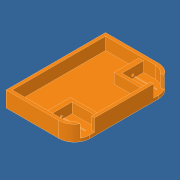
# Autodesk Inventor part: P1794_001
Saved by Autodesk Inventor 2019 (Build 230136000, 136)
## iProperties
Created: 2019-04-29
Part Number: P1794_001
Material: PLA
Document SubType Name: Modeling
Designer: Joan.MAILLARD
Density: 1.25 g/cm^3
Appearance: Orange
Project: P1704 Manette
Description: Bas manette
Author: Joan.MAILLARD
Title: P1704_001_basManette
Autodesk Inventor part; units mm, degrees
ref_plane "YZ Plane" through (0, 0, 0) normal (1, 0, 0) x (0, 1, 0)
ref_plane "XZ Plane" through (0, 0, 0) normal (0, 1, 0) x (-1, 0, 0)
ref_plane "XY Plane" through (0, 0, 0) normal (0, 0, 1) x (1, 0, 0)
sketch "Esquisse1" plane through (0, 0, 0) normal (0, 1, 0) x (-1, 0, 0)
  line L0 (55, 80) -> (55, -80)
  line L1 (-55, -80) -> (-55, 80)
  line L2 (-55, 80) -> (55, -80) construction
  line L3 (55, 80) -> (-55, -80) construction
  line L4 (0, 0) -> (-55, 0) construction
  arc A0 (-55, -55) -> (-30, -80) centre (-30, -55) ccw
  line L5 (-30, -80) -> (55, -80)
  line L6 (-30, -80) -> (-30, -55) construction
  line L7 (55, 80) -> (-30, 80)
  arc A1 (-30, 80) -> (-55, 55) centre (-30, 55) ccw
  line L8 (-30, 55) -> (-30, 80) construction
  dimension "d0" = 160
  dimension "d1" = 110
  dimension "d126" = 25
  dimension "d127" = 25
  constraints: 18 end point, 4 point on circle, 3 horizontal, 3 midpoint, 2 centre point, 2 parallel, 2 point on line, 2 tangent, 2 vertical, 1 perpendicular
  measures "d0" distance of L0.start L0.end
  measures "d1" distance of L0.end L1.start
  measures "d126" distance of L5.start L6.end
  measures "d127" distance of L8.start L7.end
extrude "Extrusion1" add sketch "Esquisse1" along normal blind 25
sketch "Esquisse2" plane through (0, 25, 0) normal (0, 1, 0) x (1, 0, 0)
  line L0 (-50, 75) -> (-50, -75)
  line L1 (-55, 80) -> (-55, -80) projected
  line L2 (30, 80) -> (-55, 80) projected
  line L3 (-50, -75) -> (30, -75)
  line L4 (30, -75) -> (30, -80) construction
  line L5 (-55, -80) -> (30, -80) construction
  line L6 (-50, 75) -> (30, 75)
  line L7 (30, 75) -> (30, 80) construction
  arc A0 (50, 55) -> (30, 75) centre (30, 55) ccw
  line L8 (30, 75) -> (30, 55) construction
  arc A1 (55, 55) -> (30, 80) centre (30, 55) ccw construction
  line L9 (50, 55) -> (50, -55)
  line L10 (55, 55) -> (50, 55) construction
  line L11 (50, -55) -> (55, -55) construction
  arc A2 (30, -75) -> (50, -55) centre (30, -55) ccw
  line L12 (55, -55) -> (55, 55) construction
  point P0 (0, 0)
  dimension "d67" = 5
  dimension "d131" = 5
  constraints: 18 end point, 4 horizontal, 4 point on circle, 3 vertical, 2 centre point, 2 tangent, 1 coincident, 1 concentric, 1 parallel, 1 perpendicular
  measures "d67" distance between parallel lines of L1 L0
  measures "d131" distance between parallel lines of L12 L9
extrude "Extrusion2" cut sketch "Esquisse2" against normal blind 20
sketch "Esquisse6" plane through (0, 5, 0) normal (0, 1, 0) x (1, 0, 0)
  line L0 (50, 40) -> (11.25, 40)
  line L1 (11.25, 40) -> (11.25, 35)
  line L2 (11.25, 35) -> (50, 35)
  line L3 (50, 35) -> (50, 40)
  line L4 (11.25, 35) -> (3.75, 35)
  line L5 (3.75, 35) -> (3.75, 75)
  line L6 (3.75, 75) -> (11.25, 75)
  line L7 (11.25, 75) -> (11.25, 35)
  line L8 (11.25, -75) -> (3.75, -75)
  line L9 (3.75, -75) -> (3.75, -35)
  line L10 (3.75, -35) -> (11.25, -35)
  line L11 (11.25, -35) -> (11.25, -75)
  line L12 (50, -35) -> (11.25, -35)
  line L13 (11.25, -35) -> (11.25, -40)
  line L14 (11.25, -40) -> (50, -40)
  line L15 (50, -40) -> (50, -35)
  line L16 (11.25, -75) -> (80.7095, -75) construction
  line L17 (50, -40) -> (50, -93.5027) construction
  line L18 (30, -75) -> (-50, -75) construction
  line L19 (50, 55) -> (50, -55) construction
  line L20 (-50, 75) -> (30, 75) construction
  point P0 (0, 0)
  point P1 (7.5, -35)
  dimension "d44" = 5
  dimension "d45" = 7.5
  dimension "d48" = 5
  dimension "d50" = 7.5
  dimension "d132" = 35
  dimension "d133" = 38.75
  dimension "d134" = 38.75
  dimension "d135" = 35
  constraints: 36 end point, 8 parallel, 5 horizontal, 5 point on line, 4 perpendicular, 1 midpoint, 1 vertical
  measures "d44" distance between parallel lines of L2 L0
  measures "d45" distance between parallel lines of L5 L7
  measures "d48" distance between parallel lines of L14 L12
  measures "d50" distance between parallel lines of L11 L9
  measures "d132" distance between parallel lines of L14 L16
  measures "d133" distance between parallel lines of L11 L17
  measures "d134" distance of L0.start L0.end
  measures "d135" distance between parallel lines of L20 L0
extrude "Extrusion4" add sketch "Esquisse6" along normal blind 16.5
sketch "Esquisse11" plane through (55, 0, 55) normal (1, 0, 0) x (0, 0, -1)
  line L0 (-12.5, 25) -> (7.5, 25)
  line L1 (7.5, 25) -> (7.5, 5)
  line L2 (7.5, 5) -> (-12.5, 5)
  line L3 (-12.5, 5) -> (-12.5, 25)
  line L4 (122.5, 25) -> (102.5, 25)
  line L5 (102.5, 25) -> (102.5, 5)
  line L6 (102.5, 5) -> (122.5, 5)
  line L7 (122.5, 5) -> (122.5, 25)
  line L8 (0, 0) -> (110, 0) projected
  line L9 (0, 25) -> (110, 25) projected
  line L10 (135, 0) -> (110, 0) projected
  line L11 (135, 25) -> (110, 25) projected
  line L12 (-25, 0) -> (-25, 25) projected
  line L13 (135, 0) -> (135, 25) projected
  line L14 (110, 5) -> (130, 5) projected
  line L15 (-20, 5) -> (0, 5) projected
  dimension "d138" = 20
  dimension "d139" = 20
  dimension "d140" = 12.5
  dimension "d141" = 12.5
  constraints: 16 end point, 4 parallel, 3 point on line, 2 horizontal, 2 perpendicular, 1 coincident, 1 midpoint
  measures "d138" distance between parallel lines of L3 L1
  measures "d139" distance between parallel lines of L7 L5
  measures "d140" distance between parallel lines of L12 L3
  measures "d141" distance between parallel lines of L13 L7
extrude "Extrusion6" cut sketch "Esquisse11" against normal blind 20
sketch "Esquisse16" plane through (11.25, 5, 75) normal (1, 0, 0) x (0, 0, -1)
  line L0 (17.5, 5) -> (7.5, 5) construction
  line L1 (17.5, 5) -> (27.5, 5) construction
  line L2 (130, 0) -> (122.5, 0) construction
  line L3 (7.5, 0) -> (7.5, 20) projected
  line L4 (27.5, 20) -> (27.5, 0) projected
  line L5 (7.5, 0) -> (20, 0) projected
  point P0 (75, -5)
  point P1 (27.5, -5)
  dimension "d137" = 5
  constraints: 4 end point, 3 point on line, 1 collinear, 1 horizontal
  measures "d137" distance between parallel lines of L5 L1
hole "Perçage6" at (11.25, 10, 57.5) direction (-1, 0, 0) diameter 3.4 depth 10
sketch "Esquisse17" plane through (11.25, 5, -40) normal (1, 0, 0) x (0, 0, -1)
  line L0 (17.5, 5) -> (7.5, 5) construction
  line L1 (17.5, 5) -> (27.5, 5) construction
  line L2 (15, 0) -> (7.5, 0) construction
  line L3 (27.5, 20) -> (27.5, 0) projected
  line L4 (7.5, 0) -> (7.5, 20) projected
  point P0 (-40, -5)
  point P1 (-87.5, 0)
  point P2 (27.5, -5)
  point P3 (7.5, -5)
  dimension "d125" = 5
  constraints: 4 end point, 2 horizontal, 2 point on line, 1 collinear
  measures "d125" distance from line of L2 L0.start
hole "Perçage7" at (11.25, 10, -57.5) direction (-1, 0, 0) diameter 3.4 depth 10
sketch "Esquisse19" plane through (0, 5, 0) normal (0, 1, 0) x (1, 0, 0)
  line L0 (45.6125, 62.1) -> (11.25, 62.1)
  line L1 (11.25, 62.1) -> (11.25, 61.1)
  line L2 (11.25, 61.1) -> (45.6125, 61.1)
  line L3 (45.6125, 61.1) -> (45.6125, 62.1)
  line L4 (45.6125, 53.9) -> (11.25, 53.9)
  line L5 (11.25, 53.9) -> (11.25, 52.9)
  line L6 (11.25, 52.9) -> (45.6125, 52.9)
  line L7 (45.6125, 52.9) -> (45.6125, 53.9)
  line L8 (50, 40) -> (11.25, 40) projected
  line L9 (45.6125, 67.5) -> (45.6125, 48.8658) construction
  line L10 (11.25, 40) -> (11.25, 75) projected
  line L11 (45.6125, -52.9) -> (11.25, -52.9)
  line L12 (11.25, -52.9) -> (11.25, -53.9)
  line L13 (11.25, -53.9) -> (45.6125, -53.9)
  line L14 (45.6125, -53.9) -> (45.6125, -52.9)
  line L15 (11.25, -61.1) -> (45.6125, -61.1)
  line L16 (45.6125, -61.1) -> (45.6125, -62.1)
  line L17 (45.6125, -62.1) -> (11.25, -62.1)
  line L18 (11.25, -62.1) -> (11.25, -61.1)
  line L19 (11.25, -40) -> (50, -40) projected
  line L20 (11.25, -75) -> (11.25, -40) projected
  point P0 (0, 0)
  dimension "d142" = 1
  dimension "d143" = 7.2
  dimension "d144" = 12.9
  dimension "d145" = 1
  dimension "d146" = 12.9
  dimension "d147" = 1
  dimension "d148" = 1
  dimension "d149" = 7.2
  constraints: 34 end point, 8 parallel, 8 point on line, 4 horizontal, 4 perpendicular, 1 coincident, 1 vertical
  measures "d142" distance between parallel lines of L2 L0
  measures "d143" distance between parallel lines of L4 L2
  measures "d144" distance between parallel lines of L8 L6
  measures "d145" distance between parallel lines of L6 L4
  measures "d146" distance between parallel lines of L19 L11
  measures "d147" distance between parallel lines of L13 L11
  measures "d148" distance between parallel lines of L17 L15
  measures "d149" distance between parallel lines of L15 L13
extrude "Extrusion11" add sketch "Esquisse19" along normal blind 0.9
equation "\"d67\" = d66"
equation "\"d131\" = d67"
equation "\"d45\" = 1.5 * d44"
equation "\"d48\" = d44"
equation "\"d50\" = d45"
equation "\"d134\" = d133"
equation "\"d135\" = d132"
equation "\"d139\" = d138"
equation "\"d141\" = d140"
equation "\"d145\" = d142"
equation "\"d146\" = d144"
equation "\"d147\" = d142"
equation "\"d148\" = d142"
equation "\"d149\" = d143"
equation "\"d66\" = 5"
